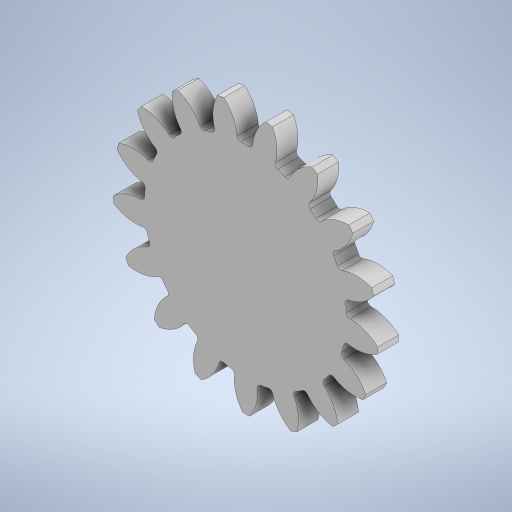
# Autodesk Inventor part: 17P_Recto
Saved by Autodesk Inventor 2023 (Build 270158030, 158C)
## iProperties
Created: 2022-05-28
Part Number: 17P_Recto
Material: Genérico
Document SubType Name: Modeling
Designer: isaac
Density: 1 g/cm^3
Appearance: Valor por defecto
Author: isaac
Autodesk Inventor part; units mm, degrees
ref_plane "YZ Plane" through (0, 0, 0) normal (1, 0, 0) x (0, 1, 0)
ref_plane "XZ Plane" through (0, 0, 0) normal (0, 1, 0) x (-1, 0, 0)
ref_plane "XY Plane" through (0, 0, 0) normal (0, 0, 1) x (1, 0, 0)
sketch "Boceto1" plane through (0, 0, 0) normal (0, 0, 1) x (1, 0, 0)
  arc A0 (188.8028, -21.2959) -> (189.622, -11.9784) centre (0, 0) ccw
  circle A1 centre (0, 0) radius 145
  arc A2 (189.622, -11.9784) -> (144.9629, 3.2779) centre (150.1138, -54.6369) ccw
  arc A3 (142.1666, -28.5247) -> (188.8028, -21.2959) centre (157.345, 27.6026) ccw
  arc A4 (183.7463, 48.3456) -> (181.1444, 57.3299) centre (0, 0) ccw
  arc A5 (181.1444, 57.3299) -> (133.9898, 55.4232) centre (159.7141, 3.2799) ccw
  arc A6 (142.8707, 24.758) -> (183.7463, 48.3456) centre (136.7486, 82.5782) ccw
  arc A7 (153.8739, 111.4577) -> (148.2022, 118.8954) centre (0, 0) ccw
  arc A8 (148.2022, 118.8954) -> (104.9206, 100.0833) centre (147.7441, 60.7538) ccw
  arc A9 (124.2794, 74.697) -> (153.8739, 111.4577) centre (97.6836, 126.4012) ccw
  arc A10 (103.2199, 159.5169) -> (95.2444, 164.4035) centre (0, 0) ccw
  arc A11 (95.2444, 164.4035) -> (61.6813, 131.2266) centre (115.8205, 110.0226) ccw
  arc A12 (88.9034, 114.5478) -> (103.2199, 159.5169) centre (45.4258, 153.153) ccw
  arc A13 (38.6256, 186.0324) -> (29.4234, 187.7079) centre (0, 0) ccw
  arc A14 (29.4234, 187.7079) -> (10.1116, 144.647) centre (68.2546, 144.4322) ccw
  arc A15 (41.5205, 138.9282) -> (38.6256, 186.0324) centre (-12.9669, 159.2206) ccw
  arc A16 (-31.1854, 187.4232) -> (-40.3714, 185.6614) centre (0, 0) ccw
  arc A17 (-40.3714, 185.6614) -> (-42.8237, 138.532) centre (11.4706, 159.3354) ccw
  arc A18 (-11.4699, 144.5456) -> (-31.1854, 187.4232) centre (-69.6084, 143.7846) ccw
  arc A19 (-96.7846, 163.5015) -> (-104.7139, 158.5402) centre (0, 0) ccw
  arc A20 (-104.7139, 158.5402) -> (-89.9755, 113.7076) centre (-46.8625, 152.7195) ccw
  arc A21 (-62.9113, 130.6414) -> (-96.7846, 163.5015) centre (-116.8489, 108.9297) ccw
  arc A22 (-149.3125, 117.498) -> (-154.9141, 110.0074) centre (0, 0) ccw
  arc A23 (-154.9141, 110.0074) -> (-124.9756, 73.5263) centre (-98.8667, 125.478) ccw
  arc A24 (-105.8562, 99.0933) -> (-149.3125, 117.498) centre (-148.3083, 59.3632) ccw
  arc A25 (-181.6749, 55.6257) -> (-184.1923, 46.6174) centre (0, 0) ccw
  arc A26 (-184.1923, 46.6174) -> (-143.097, 23.4148) centre (-137.5183, 81.29) ccw
  arc A27 (-134.5045, 54.1621) -> (-181.6749, 55.6257) centre (-159.7378, 1.7794) ccw
  arc A28 (-189.5012, -13.7591) -> (-188.5944, -23.0686) centre (0, 0) ccw
  arc A29 (-188.5944, -23.0686) -> (-141.8924, -29.8589) centre (-157.5973, 26.1233) ccw
  arc A30 (-144.9873, 1.916) -> (-189.5012, -13.7591) centre (-149.5939, -56.0447) ccw
  arc A31 (-171.7342, -81.2857) -> (-167.5257, -89.6389) centre (0, 0) ccw
  arc A32 (-167.5257, -89.6389) -> (-121.5244, -79.1001) centre (-156.392, -32.5715) ccw
  arc A33 (-135.8888, -50.5889) -> (-171.7342, -81.2857) centre (-119.2465, -106.2997) ccw
  arc A34 (-130.7736, -137.8342) -> (-123.8317, -144.1031) centre (0, 0) ccw
  arc A35 (-123.8317, -144.1031) -> (-84.7439, -117.6583) centre (-134.065, -86.8673) ccw
  arc A36 (-108.4377, -96.2614) -> (-130.7736, -137.8342) centre (-72.7942, -142.1983) ccw
  arc A37 (-72.1513, -175.7674) -> (-63.4136, -179.1053) centre (0, 0) ccw
  arc A38 (-63.4136, -179.1053) -> (-36.5182, -140.3261) centre (-93.6318, -129.4312) ccw
  arc A39 (-66.3415, -128.9333) -> (-72.1513, -175.7674) centre (-16.5106, -158.8922) ccw
  arc A40 (-3.7845, -189.9623) -> (5.5689, -189.9184) centre (0, 0) ccw
  arc A41 (5.5689, -189.9184) -> (16.6394, -144.0421) centre (-40.5531, -154.5147) ccw
  arc A42 (-15.2855, -144.1921) -> (-3.7845, -189.9623) centre (42.0028, -154.1269) ccw
  arc A43 (65.0933, -178.5017) -> (73.7992, -175.0819) centre (0, 0) ccw
  arc A44 (73.7992, -175.0819) -> (67.5498, -128.3044) centre (18.0025, -158.7301) ccw
  arc A45 (37.8348, -139.9769) -> (65.0933, -178.5017) centre (94.8435, -128.5459) ccw
  arc A46 (125.18, -142.9335) -> (132.0626, -136.5997) centre (0, 0) ccw
  arc A47 (132.0626, -136.5997) -> (109.3372, -95.2385) centre (74.1267, -141.5082) ccw
  arc A48 (85.8454, -116.857) -> (125.18, -142.9335) centre (134.8751, -85.604) ccw
  arc A49 (168.3604, -88.0613) -> (172.4902, -79.6689) centre (0, 0) ccw
  arc A50 (172.4902, -79.6689) -> (136.358, -49.3101) centre (120.2398, -105.1748) ccw
  arc A51 (122.2621, -77.955) -> (168.3604, -88.0613) centre (156.691, -31.1009) ccw
  point P0 (67.5498, -128.3044)
  point P1 (109.3372, -95.2385)
  point P2 (136.358, -49.3101)
  point P3 (142.1666, -28.5247)
  point P4 (142.8707, 24.758)
  point P5 (133.9898, 55.4232)
  point P6 (124.2794, 74.697)
  point P7 (61.6813, 131.2266)
  point P8 (-11.4699, 144.5456)
  point P9 (-42.8237, 138.532)
  point P10 (-62.9113, 130.6414)
  point P11 (-105.8562, 99.0933)
  point P12 (-134.5045, 54.1621)
  point P13 (-143.097, 23.4148)
  point P14 (-144.9873, 1.916)
  point P15 (-121.5244, -79.1001)
  point P16 (-108.4377, -96.2614)
  point P17 (-84.7439, -117.6583)
  point P18 (-36.5182, -140.3261)
  point P19 (-15.2855, -144.1921)
  point P20 (16.6394, -144.0421)
  point P21 (37.8348, -139.9769)
  dimension "d8" = 360
  constraints: 102 point on circle, 51 centre point, 3 coincident, 172 other
extrude "Extrusión1" add sketch "Boceto1" along normal blind 30
fillet "Empalme1" radius 5.235 2 edges at (41.5205, 138.9282, 15) (61.6813, 131.2266, 15)
pattern_circular "Patrón circular1" count 17 over 360 about axis through (0, 0, 0) along (0, 0, 1) of "Empalme1"
